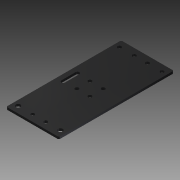
# Autodesk Inventor part: x-carriage
Saved by Autodesk Inventor 2014 (Build 180170000, 170)
## iProperties
Created: 2013-07-12
Part Number: x-carriage
Material: Steel, Mild
Document SubType Name: Modeling
Designer: Edward
Density: 7.86 g/cm^3
Appearance: Lacquer - Black
Author: Edward
Autodesk Inventor part; units mm, degrees
ref_plane "YZ Plane" through (0, 0, 0) normal (1, 0, 0) x (0, 1, 0)
ref_plane "XZ Plane" through (0, 0, 0) normal (0, 1, 0) x (-1, 0, 0)
ref_plane "XY Plane" through (0, 0, 0) normal (0, 0, 1) x (1, 0, 0)
sketch "Sketch1" plane through (0, 0, 0) normal (0, 0, 1) x (1, 0, 0)
  line L0 (-40, 87.5) -> (40, 87.5)
  line L1 (40, 87.5) -> (40, -87.5)
  line L2 (40, -87.5) -> (-40, -87.5)
  line L3 (-40, -87.5) -> (-40, 87.5)
  point P0 (0, 0)
  dimension "d0" = 80
  dimension "d1" = 175
  dimension "d2" = 40
  dimension "d3" = 87.5
  constraints: 8 end point, 2 parallel, 1 horizontal, 1 perpendicular
  measures "d0" distance of L1.end L2.end
  measures "d1" distance of L0.end L1.end
  measures "d2" distance from line of point (0, 0) L3
  measures "d3" distance from line of L0 point (0, 0)
extrude "Extrusion1" add sketch "Sketch1" along normal blind 3.4163
sketch "Sketch2" plane through (0, 0, 3.4163) normal (0, 0, 1) x (1, 0, 0)
  line L0 (40, 87.5) -> (-40, 87.5) projected
  line L1 (-40, 87.5) -> (-40, -87.5) projected
  circle A0 centre (-32.3, 77.3) radius 2.75
  circle A1 centre (32.3, 77.3) radius 2.75
  point P0 (0, 0)
  dimension "d6" = 5.5
  dimension "d7" = 10.2
  dimension "d12" = 5.5
  dimension "d13" = 64.6
  dimension "d14" = 7.7
  dimension "d15" = 10.2
  constraints: 2 centre point
  measures "d6" diameter of A0
  measures "d7" distance from line of L0 A0.centre
  measures "d12" diameter of A1
  measures "d13" distance of A0.centre A1.centre
  measures "d14" distance from line of L1 A0.centre
  measures "d15" distance from line of L0 A1.centre
extrude "Extrusion2" cut sketch "Sketch2" against normal through all
pattern_linear "Rectangular Pattern1" count 2 spacing 154.6 along (0, -1, 0) of "Extrusion2"
sketch "Sketch3" plane through (0, 0, 3.4163) normal (0, 0, 1) x (1, 0, 0)
  line L0 (40, 87.5) -> (-40, 87.5) projected
  line L1 (-40, 87.5) -> (-40, -87.5) projected
  line L2 (-30, 11) -> (-30, -11) construction
  line L3 (-32.75, 11) -> (-32.75, -11)
  line L4 (-27.25, -11) -> (-27.25, 11)
  arc A0 (-27.25, 11) -> (-32.75, 11) centre (-30, 11) ccw
  arc A1 (-32.75, -11) -> (-27.25, -11) centre (-30, -11) ccw
  point P0 (0, 0)
  point P1 (-30, 0)
  dimension "d25" = 22
  dimension "d26" = 5.5
  dimension "d27" = 76.5
  dimension "d35" = 10
  constraints: 8 end point, 4 point on circle, 4 tangent, 2 centre point, 2 parallel, 1 midpoint
  measures "d25" distance of L2.start L2.end
  measures "d26" diameter of A1
  measures "d27" distance from line of L0 L2.start
  measures "d35" distance from line of L1 L2.start
extrude "Extrusion3" cut sketch "Sketch3" against normal through all
sketch "Sketch4" plane through (0, 0, 3.4163) normal (0, 0, 1) x (1, 0, 0)
  circle A0 centre (-32.3, -77.3) radius 2.75 projected
  circle A1 centre (32.3, -77.3) radius 2.75 projected
  circle A2 centre (-32.3, -77.3) radius 3.58
  circle A3 centre (32.3, -77.3) radius 3.58
  point P0 (0, 0)
  dimension "d31" = 7.16
  dimension "d32" = 7.16
  constraints: 2 centre point, 2 coincident
  measures "d31" diameter of A2
  measures "d32" diameter of A3
extrude "Extrusion4" cut sketch "Sketch4" against normal through all
fillet "Fillet1" radius 2 4 edges at (40, 87.5, 1.7082) (-40, 87.5, 1.7082) (-40, -87.5, 1.7082) (40, -87.5, 1.7082)
sketch "Sketch5" plane through (0, 0, 3.4163) normal (0, 0, 1) x (1, 0, 0)
  line L0 (38, 87.5) -> (-38, 87.5) projected
  line L1 (-40, 85.5) -> (-40, -85.5) projected
  circle A0 centre (-10, 77.5) radius 2.75
  line L2 (-38, -87.5) -> (38, -87.5) projected
  circle A1 centre (-10, 10) radius 2.75
  circle A2 centre (-10, -10) radius 2.75
  circle A3 centre (-10, -77.5) radius 2.75
  point P0 (0, 0)
  dimension "d37" = 5.5
  dimension "d38" = 30
  dimension "d39" = 10
  dimension "d48" = 5.5
  dimension "d49" = 77.5
  dimension "d50" = 5.5
  dimension "d51" = 97.5
  dimension "d52" = 5.5
  dimension "d53" = 10
  dimension "d54" = 30
  dimension "d55" = 30
  dimension "d56" = 30
  constraints: 4 centre point
  measures "d37" diameter of A0
  measures "d38" distance from line of L1 A0.centre
  measures "d39" distance from line of L0 A0.centre
  measures "d48" diameter of A1
  measures "d49" distance from line of L0 A1.centre
  measures "d50" diameter of A2
  measures "d51" distance from line of L0 A2.centre
  measures "d52" diameter of A3
  measures "d53" distance from line of L2 A3.centre
  measures "d54" distance from line of L1 A3.centre
  measures "d55" distance from line of L1 A2.centre
  measures "d56" distance from line of L1 A1.centre
extrude "Extrusion5" cut sketch "Sketch5" against normal through all
pattern_linear "Rectangular Pattern3" count 2 spacing 20 along (1, 0, 0) of "Extrusion5"
equation "\"d2\" = 0.5 * d0"
equation "\"d3\" = 0.5 * d1"
equation "\"d15\" = d7"
body "Solid1"
